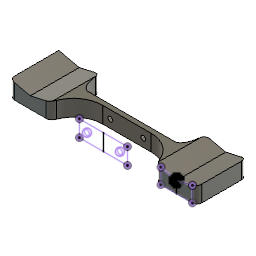
TorqueCalibrationArm (Autodesk Fusion 360 design; units mm, degrees)
Autodesk Fusion 360 part; units mm, degrees
sketch "Sketch1" plane through (0, 0, 0) normal (0, 0, 1) x (1, 0, 0)
  line L0 (-21.1, 7) -> (21.1, 7)
  line L1 (21.1, 7) -> (21.1, -7)
  line L2 (21.1, -7) -> (-21.1, -7)
  line L3 (-21.1, -7) -> (-21.1, 7)
  circle A0 centre (-14.1, 0) radius 2.075
  circle A1 centre (14.1, 0) radius 2.075
  line L4 (-14.1, 0) -> (14.1, 0) construction
  line L5 (-21.1, 0) -> (21.1, 0) construction
  line L6 (21.1, 7) -> (45.1, 7)
  line L7 (45.1, 7) -> (45.1, -7) construction
  line L8 (45.1, -7) -> (21.1, -7)
  line L9 (-21.1, -7) -> (-21.1, 7)
  line L10 (45.1, 7) -> (62.6, 3)
  line L11 (62.6, 3) -> (80.1, 7)
  line L12 (45.1, -7) -> (80.1, -7)
  line L13 (80.1, -7) -> (80.1, 7)
  line L14 (0, 7) -> (0, -7) construction
  line L15 (-21.1, 7) -> (-45.1, 7)
  line L16 (-45.1, 7) -> (-62.6, 3)
  line L17 (-62.6, 3) -> (-80.1, 7)
  line L18 (-80.1, -7) -> (-80.1, 7)
  line L19 (-45.1, -7) -> (-80.1, -7)
  line L20 (-45.1, -7) -> (-21.1, -7)
  dimension "d1" = 28.2
  dimension "d2" = 4.15
  dimension "d4" = 7
  dimension "d5" = 7
  dimension "d8" = 24
  dimension "d9" = 10
  dimension "d10" = 35
  constraint horizontal L0
  constraint vertical L1
  constraint horizontal L2
  constraint vertical L3
  constraint equal A0 A1
  constraint coincident A0.centre L4.start
  constraint coincident A1.centre L4.end
  constraint midpoint L4 origin
  constraint midpoint L3 L5.start
  constraint midpoint L1 L5.end
  constraint midpoint L5 origin
  constraint collinear L4 L5
  constraint horizontal L6
  constraint vertical L7
  constraint horizontal L8
  constraint coincident L0.end L1.start
  constraint coincident L1.end L2.start
  constraint vertical L9
  constraint coincident L2.end L3.start
  constraint perpendicular L7 L12
  constraint vertical L13
  constraint equal L7 L13
  constraint equal L10 L11
  constraint midpoint L0 L14.start
  constraint midpoint L2 L14.end
  constraint symmetric L0.end L14 L0.start
  constraint symmetric L6.end L14 L15.end
  constraint symmetric L7.end L14 L19.start
  constraint symmetric L1.end L14 L2.end
  constraint symmetric L10.end L14 L16.end
  constraint symmetric L11.end L14 L17.end
  constraint symmetric L12.end L14 L18.start
  measures "d1" distance of A0.centre A1.centre
  measures "d2" diameter of A0
  measures "d4" distance of L0 A0.centre
  measures "d5" distance of L3 A0.centre
  measures "d8" distance of L0.end L6.end
  measures "d9" distance of L10.end L12
  measures "d10" distance of L7 L13
extrude "Extrude1" add sketch "Sketch1" along normal blind 4
sketch "Sketch2" plane through (0, 0, 4) normal (0, 0, 1) x (1, 0, 0)
  circle A0 centre (-14.1, 0) radius 2.075
  circle A1 centre (14.1, 0) radius 2.075
  line L0 (-80.1, -7) -> (80.1, -7)
  line L1 (80.1, -7) -> (80.1, 7)
  line L2 (80.1, 7) -> (62.6, 3)
  line L3 (62.6, 3) -> (45.1, 7)
  line L4 (45.1, 7) -> (-45.1, 7)
  line L5 (-45.1, 7) -> (-62.6, 3)
  line L6 (-62.6, 3) -> (-80.1, 7)
  line L7 (-80.1, 7) -> (-80.1, -7)
  line L8 (-45.1, 7) -> (-45.1, -7)
  line L9 (-45.1, 7) -> (-62.6, 3)
  line L10 (-62.6, 3) -> (-80.1, 7)
  line L11 (-80.1, 7) -> (-80.1, -7)
  line L12 (-45.1, -7) -> (-80.1, -7)
  line L13 (80.1, -7) -> (80.1, 7)
  line L14 (80.1, 7) -> (62.6, 3)
  line L15 (45.1, 7) -> (62.6, 3)
  line L16 (45.1, 7) -> (45.1, -7)
  line L17 (80.1, -7) -> (45.1, -7)
  constraint coincident L4.end L5.start
  constraint coincident L0 L8.end
  constraint perpendicular L0 L8
  constraint coincident L5.end L6.start
  constraint coincident L6.end L7.start
  constraint coincident L0.start L7.end
  constraint coincident L0.end L1.start
  constraint coincident L1.end L2.start
  constraint coincident L2.end L3.start
  constraint coincident L3.end L4.start
  constraint coincident L0 L16.end
  constraint perpendicular L0 L16
extrude "Extrude2" add sketch "Sketch2" along normal blind 20 and the other way blind 22 contours L0 L5 L6 L7 L8 L9 L10 L11 L12 | L0 L1 L2 L3 L13 L14 L15 L16 L17
fillet "Fillet1" radius 25 2 edges at (-45.1, 0, 4) (45.1, 0, 4)
fillet "Fillet2" offset 8 second offset 18 1 edges at (45.1, 0, 0) measured on face at (-35.4583, 0, 0)
fillet "Fillet3" offset 8 second offset 18 1 edges at (-45.1, 0, 0) measured on face at (-35.4583, 0, 0)
fillet "Fillet4" offset 4 second offset 4 7 edges at (45.1, 0, -18) (-45.1, 0, -18) (80.1, 0, -18) (-80.1, 0, 24) (-45.1, 0, 24) (45.1, 0, 24) (80.1, 0, 24) measured on face at (50.9333, 1, -18) measured on face at (-50.9333, 1, -18) measured on face at (50.9333, 1, -18) measured on face at (-50.9333, 1, 24) measured on face at (-50.9333, 1, 24) measured on face at (50.9333, 1, 24) measured on face at (50.9333, 1, 24)
sketch "Sketch4" plane through (0, 0, 24) normal (0, 0, 1) x (1, 0, 0)
  line L0 (-49.1, 6.0857) -> (-49.1, -7)
  line L1 (-49.1, 6.0857) -> (-62.6, 3)
  line L2 (-62.6, 3) -> (-76.1, 6.0857)
  line L3 (-76.1, -7) -> (-76.1, 6.0857)
  line L4 (-76.1, -7) -> (-49.1, -7)
  line L5 (20.6051, -7) -> (20.6051, 7)
  line L6 (20.6051, 7) -> (-20.6051, 7)
  line L7 (-20.6051, 7) -> (-20.6051, -7)
  line L8 (-20.6051, -7) -> (20.6051, -7)
  circle A0 centre (14.1, 0) radius 2.075
  circle A1 centre (-14.1, 0) radius 2.075
  line L9 (76.1, 6.0857) -> (76.1, -7)
  line L10 (76.1, 6.0857) -> (62.6, 3)
  line L11 (62.6, 3) -> (49.1, 6.0857)
  line L12 (49.1, -7) -> (49.1, 6.0857)
  line L13 (49.1, -7) -> (76.1, -7)
  line L14 (0, 7) -> (0, -7)
  line L15 (62.6, 3) -> (62.6, -7)
  constraint midpoint L6 L14.start
  constraint midpoint L8 L14.end
  constraint coincident L10.end L11.start
  constraint midpoint L13 L15.end
equation "d2 = 4 mm + hole_tolerance"
equation "hole_tolerance = 0.15 mm"
